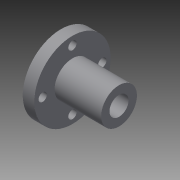
# Autodesk Inventor part: linear bearing
Saved by Autodesk Inventor 2015 SP1 (Build 190203100, 203)
## iProperties
Created: 2016-07-11
Part Number: linear bearing
Material: Generic
Document SubType Name: Modeling
Designer: lustinga
Density: 1 g/cm^3
Appearance: Default
Mass: 5.92161 g
Surface Area: 36.5939 cm^2
Volume: 5.92161 cm^3
Author: lustinga
Autodesk Inventor part; units mm, degrees
ref_plane "YZ Plane" through (0, 0, 0) normal (1, 0, 0) x (0, 1, 0)
ref_plane "XZ Plane" through (0, 0, 0) normal (0, 1, 0) x (-1, 0, 0)
ref_plane "XY Plane" through (0, 0, 0) normal (0, 0, 1) x (1, 0, 0)
sketch "Sketch1" plane through (0, 0, 0) normal (1, 0, 0) x (0, 1, 0)
  circle A0 centre (0, 0) radius 16
  circle A1 centre (-12, 0) radius 1.75
  circle A2 centre (0, -12) radius 1.75
  circle A3 centre (12, 0) radius 1.75
  circle A4 centre (0, 12) radius 1.75
  circle A5 centre (0, 0) radius 7.5
  circle A6 centre (0, 0) radius 4
  dimension "d0" = 32
  dimension "d1" = 3.5
  dimension "d4" = 360
  dimension "d6" = 24
  dimension "d7" = 15
  dimension "d8" = 8
  dimension "d14" = 12
  constraints: 7 centre point, 2 coincident, 9 other
  measures "d0" diameter of A0
  measures "d1" diameter of A1
  measures "d6" distance of A3.centre A1.centre
  measures "d7" diameter of A5
  measures "d8" diameter of A6
  measures "d14" distance of A6.centre A2.centre
extrude "Extrusion1" add sketch "Sketch1" along normal blind 4.83 contours A0 | A5
sketch "Sketch2" plane through (4.83, 0, 0) normal (1, 0, 0) x (0, 0, -1)
  circle A0 centre (0, 0) radius 4 projected
  circle A1 centre (0, 0) radius 7.5
  point P0 (0, 0)
  dimension "d11" = 15
  constraints: 1 centre point, 1 coincident
  measures "d11" diameter of A1
extrude "Extrusion2" add sketch "Sketch2" along normal blind 19.5
body "Solid1"
